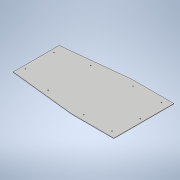
# Autodesk Inventor part: frontfloorfit2
Saved by Autodesk Inventor 2021 (Build 250183000, 183)
## iProperties
Created: 2020-10-26
Part Number: frontfloorfit2
Material: Generic
Document SubType Name: Modeling
Designer: mackeycj
Density: 1 g/cm^3
Appearance: Default
Author: mackeycj
Autodesk Inventor part; units mm, degrees
ref_plane "YZ Plane" through (0, 0, 0) normal (1, 0, 0) x (0, 1, 0)
ref_plane "XZ Plane" through (0, 0, 0) normal (0, 1, 0) x (-1, 0, 0)
ref_plane "XY Plane" through (0, 0, 0) normal (0, 0, 1) x (1, 0, 0)
sketch "Sketch1" plane through (0, 0, 0) normal (0, 1, 0) x (-1, 0, 0)
  line L0 (0, 0) -> (0, 215.9)
  line L1 (0, 215.9) -> (304.8, 215.9)
  line L2 (0, 0) -> (774.7, 0)
  line L3 (0, 0) -> (0, -215.9)
  line L4 (0, -215.9) -> (304.8, -215.9)
  line L5 (774.7, 0) -> (774.7, -165.1)
  line L6 (774.7, -165.1) -> (774.7, 0)
  line L7 (774.7, 0) -> (774.7, 165.1)
  line L8 (774.7, 165.1) -> (304.8, 215.9)
  line L9 (774.7, -165.1) -> (304.8, -215.9)
  line L10 (0, -215.9) -> (50.8, -215.9)
  line L11 (50.8, -215.9) -> (50.8, -177.8)
  line L12 (304.8, -215.9) -> (254, -215.9)
  line L13 (254, -215.9) -> (254, -177.8)
  line L14 (539.75, -190.5) -> (535.6549, -152.6207)
  line L15 (774.7, 0) -> (774.7, -101.6)
  line L16 (774.7, -101.6) -> (749.3, -101.6)
  line L17 (774.7, 0) -> (774.7, 101.6)
  line L18 (774.7, 101.6) -> (749.3, 101.6)
  circle A0 centre (749.3, 101.6) radius 3.175
  circle A1 centre (749.3, -101.6) radius 3.175
  line L19 (539.75, 190.5) -> (535.6549, 152.6207)
  circle A2 centre (535.6549, 152.6207) radius 3.175
  line L20 (0, 215.9) -> (50.8, 215.9)
  line L21 (50.8, 215.9) -> (50.8, 177.8)
  line L22 (304.8, 215.9) -> (254, 215.9)
  line L23 (254, 215.9) -> (254, 177.8)
  circle A3 centre (254, 177.8) radius 3.175
  circle A4 centre (50.8, 177.8) radius 3.175
  circle A5 centre (50.8, -177.8) radius 3.175
  circle A6 centre (254, -177.8) radius 3.175
  circle A7 centre (535.6549, -152.6207) radius 3.175
  line L24 (0, 0) -> (25.4, 0)
  circle A8 centre (25.4, 0) radius 3.175
  dimension "d0" = 215.9
  dimension "d1" = 304.8
  dimension "d2" = 774.7
  dimension "d3" = 215.9
  dimension "d4" = 304.8
  dimension "d5" = 165.1
  dimension "d6" = 165.1
  dimension "d9" = 50.8
  dimension "d10" = 38.1
  dimension "d11" = 50.8
  dimension "d12" = 38.1
  dimension "d14" = 38.1
  dimension "d15" = 101.6
  dimension "d16" = 25.4
  dimension "d17" = 101.6
  dimension "d18" = 25.4
  dimension "d19" = 6.35
  dimension "d20" = 6.35
  dimension "d21" = 38.1
  dimension "d22" = 6.35
  dimension "d23" = 50.8
  dimension "d24" = 38.1
  dimension "d25" = 50.8
  dimension "d26" = 38.1
  dimension "d27" = 6.35
  dimension "d28" = 6.35
  dimension "d29" = 6.35
  dimension "d30" = 6.35
  dimension "d31" = 6.35
  dimension "d32" = 25.4
  dimension "d33" = 6.35
  constraints: 50 end point, 11 perpendicular, 9 centre point, 9 coincident, 7 point on line, 3 vertical, 2 midpoint, 1 collinear, 1 horizontal
  measures "d0" distance of L0.start L0.end
  measures "d1" distance of L0.end L1.end
  measures "d2" distance of L0.start L2.end
  measures "d3" distance of L0.start L3.end
  measures "d4" distance of L3.end L4.end
  measures "d5" distance of L2.end L5.end
  measures "d6" distance of L2.end L7.end
  measures "d9" distance of L3.end L10.end
  measures "d10" distance of L10.end L11.end
  measures "d11" distance of L4.end L12.end
  measures "d12" distance of L12.end L13.end
  measures "d14" distance of L14.start L14.end
  measures "d15" distance of L2.end L15.end
  measures "d16" distance of L15.end L16.end
  measures "d17" distance of L2.end L17.end
  measures "d18" distance of L17.end L18.end
  measures "d19" diameter of A0
  measures "d20" diameter of A1
  measures "d21" distance of L19.start L19.end
  measures "d22" diameter of A2
  measures "d23" distance of L0.end L20.end
  measures "d24" distance of L20.end L21.end
  measures "d25" distance of L1.end L22.end
  measures "d26" distance of L22.end L23.end
  measures "d27" diameter of A3
  measures "d28" diameter of A4
  measures "d29" diameter of A5
  measures "d30" diameter of A6
  measures "d31" diameter of A7
  measures "d32" distance of L0.start L24.end
  measures "d33" diameter of A8
extrude "Extrusion1" add sketch "Sketch1" along normal blind 3.175 contours L0 L1 L8 L7 L2 A8 | L2 A8 L5 L9 L4 L3
body "Solid1"
